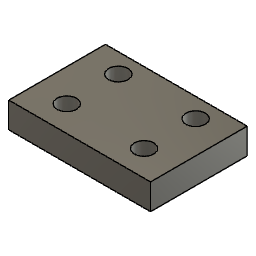
braçadeira v2 (Autodesk Fusion 360 design; units mm, degrees)
Autodesk Fusion 360 part; units mm, degrees
sketch "Sketch1" plane through (0, 0, 0) normal (0, 1, 0) x (1, 0, 0)
  line L0 (0, 0) -> (22, 0)
  line L1 (22, 0) -> (22, -15)
  line L2 (22, -15) -> (0, -15)
  line L3 (0, -15) -> (0, 0)
  circle A0 centre (17, -11) radius 1.5
  line L4 (0, -15) -> (0, -14.748)
  circle A1 centre (5, -3) radius 1.5
  circle A2 centre (17, -3) radius 1.5
  circle A3 centre (5, -11) radius 1.5
  dimension "d11" = 3
  dimension "d18" = 3
  dimension "d21" = 3
  dimension "d24" = 3
  constraint horizontal L0
  constraint vertical L1
  constraint horizontal L2
  constraint vertical L3
  constraint coincident L0.start L3.end
  constraint coincident L3 L4.end
  measures "d11" diameter of A0
  measures "d18" diameter of A1
  measures "d21" diameter of A2
  measures "d24" diameter of A3
extrude "Extrude1" add sketch "Sketch1" along normal blind 4 makes body 1
copy_body "Body->Comp1" bodies 1 removing the originals makes body 2 in component "Component"
component "Component" placed x (1, 0, 0) y (0, 1, 0) z (0, 0, 1) at (0, 0, 0)
